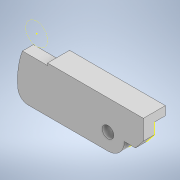
# Autodesk Inventor part: Capping_RotationGuide
Saved by Autodesk Inventor 2022 (Build 260153000, 153)
## iProperties
Created: 2024-05-21
Part Number: Capping_RotationGuide
Material: Generic
Document SubType Name: Modeling
Designer: Gotham City
Density: 1 g/cm^3
Appearance: Default
Author: Gotham City
Autodesk Inventor part; units mm, degrees
ref_plane "YZ Plane" through (0, 0, 0) normal (1, 0, 0) x (0, 1, 0)
ref_plane "XZ Plane" through (0, 0, 0) normal (0, 1, 0) x (-1, 0, 0)
ref_plane "XY Plane" through (0, 0, 0) normal (0, 0, 1) x (1, 0, 0)
sketch "Sketch1" plane through (0, 0, 0) normal (0, 0, 1) x (1, 0, 0)
  circle A0 centre (4.056, -0.4) radius 1.05 projected
  line L0 (-10.5, -3.4) -> (-10.5, 3.4) projected
  line L1 (4.056, -3.4) -> (-10.5, -3.4) projected
  arc A1 (4.056, -3.4) -> (7.056, -0.4) centre (4.056, -0.4) ccw projected
  line L2 (9.056, -0.4) -> (7.056, -0.4) projected
  line L3 (10.5, 1.4) -> (9.056, -0.4) projected
  line L4 (10.5, 3.4) -> (10.5, 1.4) projected
  line L5 (-10.5, 3.4) -> (10.5, 3.4) projected
  point P0 (0, 0)
sketch "Sketch2" plane through (0, 0, 0) normal (0, 0, 1) x (1, 0, 0)
  arc A0 (-11.5298, 4.6) -> (-12.3624, -1.6977) centre (2.056, -0.4) ccw
  line L0 (4.056, -0.4) -> (2.056, -0.4) construction
  circle A1 centre (-10.944, 6.6) radius 2 construction
  line L1 (-11.5298, 4.6) -> (-8.944, 4.6)
  line L2 (-11.5298, 4.6) -> (4.056, -0.4) construction
  line L3 (4.056, -0.4) -> (-12.3624, -1.6977) construction
  circle A2 centre (-12.944, 6.0142) radius 2 construction
  line L4 (-12.944, 6.0142) -> (-11.5298, 4.6) construction
  line L5 (-12.944, 6.0142) -> (-10.944, 6.0142) construction
  line L6 (4.056, -3.4) -> (-10.5, -3.4) construction
  arc A3 (-12.3624, -1.6977) -> (-10.5, -3.4) centre (-10.5, -1.5301) ccw
  point P0 (0, 0)
  point P1 (-8.944, 6.6)
  dimension "d1" = 4
  dimension "d0" = 2
  dimension "d2" = 7
  dimension "d3" = 15
  dimension "d11" = 45
  dimension "d12" = 2
  constraints: 12 end point, 6 point on circle, 4 horizontal, 3 centre point, 2 horizontal alignment, 2 tangent, 1 coincident, 1 vertical alignment, 3 other
  measures "d0" distance of L0.start L0.end
  measures "d2" vertical distance of L0.start point (-10.944, 6.6)
  measures "d3" horizontal distance of point (-10.944, 6.6) L0.start
  measures "d11" angle of L4 L5
  measures "d12" horizontal distance of L4.start point (-10.944, 6.6)
sketch "Sketch3" plane through (0, 0, 0) normal (0, 0, 1) x (1, 0, 0)
  arc A0 (-11.5298, 4.6) -> (-12.3624, -1.6977) centre (2.056, -0.4) ccw projected
  line L0 (-11.5298, 4.6) -> (-8.944, 4.6) projected
  line L1 (10.5, 5) -> (10.5, 1.4)
  line L2 (10.5, 3.4) -> (10.5, 1.4) construction
  circle A1 centre (4.056, -0.4) radius 1.05 projected
  line L3 (4.056, -3.4) -> (-10.5, -3.4) projected
  arc A2 (4.056, -3.4) -> (7.056, -0.4) centre (4.056, -0.4) ccw projected
  line L4 (9.056, -0.4) -> (7.056, -0.4) projected
  line L5 (10.5, 1.4) -> (9.056, -0.4) projected
  arc A3 (-12.3624, -1.6977) -> (-10.5, -3.4) centre (-10.5, -1.5301) ccw projected
  line L6 (-8.944, 4.6) -> (-6.944, 4.6)
  line L7 (-6.944, 4.6) -> (-6.944, 5)
  line L8 (-6.944, 5) -> (10.5, 5)
  line L9 (-10.5, 3.4) -> (10.5, 3.4) construction
  point P0 (0, 0)
  dimension "d18" = 1.6
  dimension "d19" = 2
  constraints: 8 end point, 2 perpendicular, 1 horizontal, 1 point on line
  measures "d18" distance between parallel lines of L8 L9
  measures "d19" distance of L0.end L6.end
extrude "Extrusion1" add sketch "Sketch3" along normal blind 2
sketch "Sketch4" plane through (0, 0, 0) normal (0, 0, -1) x (-1, 0, 0)
  arc A0 (12.3624, -1.6977) -> (11.5298, 4.6) centre (-2.056, -0.4) ccw projected
  line L0 (6.944, 4.6) -> (11.5298, 4.6) projected
  line L1 (-10.5, 1.4) -> (-10.5, 5) projected
  line L2 (-9.056, -0.4) -> (-10.5, 1.4) projected
  line L3 (-7.056, -0.4) -> (-9.056, -0.4) projected
  arc A1 (-7.056, -0.4) -> (-4.056, -3.4) centre (-4.056, -0.4) ccw projected
  line L4 (10.5, -3.4) -> (-4.056, -3.4) projected
  arc A2 (10.5, -3.4) -> (12.3624, -1.6977) centre (10.5, -1.5301) ccw projected
  circle A3 centre (-4.056, -0.4) radius 1.05 projected
  line L5 (6.944, 5) -> (6.944, 4.6) projected
  line L6 (-10.5, 5) -> (6.944, 5) projected
  line L7 (-10.5, 5) -> (6.944, 5) projected
  line L8 (-10.5, 1.4) -> (-10.5, 5) projected
  line L9 (6.944, 5) -> (-10.5, 5)
  line L10 (-10.5, 5) -> (-10.5, 3.4)
  line L11 (-10.5, 3.4) -> (6.944, 3.4)
  line L12 (6.944, 3.4) -> (6.944, 5)
  line L13 (-10.5, 1.4) -> (-10.5, 5) projected
  constraints: 8 end point, 2 parallel, 1 horizontal, 1 perpendicular, 1 point on line
extrude "Extrusion2" add sketch "Sketch4" along normal blind 2 contours L12 L11 L1 L6 L5
sketch "Sketch5" plane through (0, 0, 0) normal (0, 0, 1) x (1, 0, 0)
  circle A0 centre (-10.944, 6.6) radius 2 construction
  point P0 (0, 0)
equation "\"d12\" = d0"
body "Solid1"
